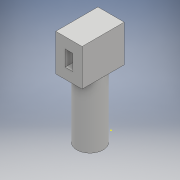
# Autodesk Inventor part: 武士刀夾具
Saved by Autodesk Inventor 2017 (Build 210142000, 142)
## iProperties
Created: 2021-05-18
Part Number: 武士刀夾具
Material: Generic
Document SubType Name: Modeling
Designer: user
Density: 1 g/cm^3
Appearance: Default
Author: user
Autodesk Inventor part; units mm, degrees
ref_plane "YZ Plane" through (0, 0, 0) normal (1, 0, 0) x (0, 1, 0)
ref_plane "XZ Plane" through (0, 0, 0) normal (0, 1, 0) x (-1, 0, 0)
ref_plane "XY Plane" through (0, 0, 0) normal (0, 0, 1) x (1, 0, 0)
sketch "Sketch1" plane through (0, 0, 0) normal (0, 0, 1) x (1, 0, 0)
  circle A0 centre (0, 0) radius 25
  dimension "d0" = 50
  constraints: 1 centre point, 1 coincident
  measures "d0" diameter of A0
extrude "Extrusion1" add sketch "Sketch1" along normal blind 120
sketch "Sketch5" plane through (0, 0, 120) normal (0, 0, 1) x (1, 0, 0)
  line L0 (-25, -40) -> (25, -40)
  line L1 (25, -40) -> (25, 40)
  line L2 (25, 40) -> (-25, 40)
  line L3 (-25, 40) -> (-25, -40)
  line L4 (-25, -40) -> (25, 40) construction
  line L5 (25, -40) -> (-25, 40) construction
  point P0 (0, 0)
  dimension "d18" = 50
  dimension "d19" = 80
  constraints: 12 end point, 2 midpoint, 2 parallel, 1 horizontal, 1 perpendicular
  measures "d18" distance of L1.end L2.end
  measures "d19" distance of L2.end L0.start
extrude "Extrusion4" add sketch "Sketch5" along normal blind 70
sketch "Sketch6" plane through (-25, 40, 120) normal (0, 1, 0) x (1, 0, 0)
  point P0 (25, 120)
sketch "Sketch7" plane through (-25, 40, 120) normal (0, 1, 0) x (1, 0, 0)
  line L0 (0, 0) -> (50, 0) projected
  line L1 (0, -70) -> (50, -70) projected
  line L2 (50, 0) -> (0, -70)
  line L3 (32.1175, -49.918) -> (17.8825, -49.918)
  line L4 (17.8825, -49.918) -> (17.8825, -20.082)
  line L5 (17.8825, -20.082) -> (32.1175, -20.082)
  line L6 (32.1175, -20.082) -> (32.1175, -49.918)
  line L7 (32.1175, -49.918) -> (17.8825, -20.082) construction
  line L8 (17.8825, -49.918) -> (32.1175, -20.082) construction
  point P0 (25, 120)
  point P1 (25, -35)
  dimension "d22" = 14.235
  dimension "d23" = 29.836
  constraints: 14 end point, 3 midpoint, 2 parallel, 1 horizontal, 1 perpendicular
  measures "d22" distance of L4.end L5.end
  measures "d23" distance of L3.end L4.end
extrude "Extrusion5" cut sketch "Sketch7" against normal through all
body "Solid1"
